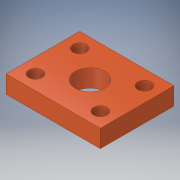
# Autodesk Inventor part: Hopper Nut Trap Holder
Saved by Autodesk Inventor 2018 (Build 220112000, 112)
## iProperties
Created: 2013-10-19
Part Number: Hopper Nut Trap Holder
Material: ABS Plastic
Document SubType Name: Modeling
Designer: Gabriel Smolnycki
Mass: 4.18388 g
Surface Area: 25.2747 cm^2
Volume: 3.94706 cm^3
Density: 1.06 g/cm^3
Appearance: Smooth - Light Orange
Sending System: SolidWorks 2017
Last Author: Gabriel Smolnycki
Last Saved: 2017-09-14
Author: Gabriel Smolnycki
Autodesk Inventor part; units mm, degrees
ref_plane "YZ Plane" through (0, 0, 0) normal (1, 0, 0) x (0, 1, 0)
ref_plane "XZ Plane" through (0, 0, 0) normal (0, 1, 0) x (-1, 0, 0)
ref_plane "XY Plane" through (0, 0, 0) normal (0, 0, 1) x (1, 0, 0)
sketch "Sketch1" plane through (0, 0, 0) normal (0, 1, 0) x (-1, 0, 0)
  line L0 (-16, 12.5) -> (-16, -12.5)
  line L1 (16, 12.5) -> (-16, 12.5)
  line L2 (16, -12.5) -> (16, 12.5)
  line L3 (-16, -12.5) -> (16, -12.5)
  constraints: 8 end point, 2 horizontal, 2 vertical
extrude "Extrusion1" add sketch "Sketch1" along normal blind 6
hole "Hole5" at (0, 6, 0) direction (0, -1, 0) diameter 10 depth 6 tip angle 118
hole "Hole4" at (-11, 6, -7.5) direction (0, -1, 0) diameter 4.5 depth 6 tip angle 118
sketch "Sketch4" plane through (0, 6, 0) normal (0, 1, 0) x (1, 0, 0)
  point P0 (11, -7.5)
hole "Hole3" at (11, 6, 7.5) direction (0, -1, 0) diameter 4.5 depth 6 tip angle 118
sketch "Sketch3" plane through (0, 6, 0) normal (0, 1, 0) x (1, 0, 0)
  point P0 (-11, 7.5)
hole "Hole2" at (11, 6, -7.5) direction (0, -1, 0) diameter 4.5 depth 6 tip angle 118
sketch "Sketch2" plane through (0, 6, 0) normal (0, 1, 0) x (1, 0, 0)
  point P0 (0, 0)
hole "Hole1" at (-11, 6, 7.5) direction (0, -1, 0) diameter 4.5 depth 6 tip angle 118
sketch "Sketch5" plane through (0, 6, 0) normal (0, 1, 0) x (1, 0, 0)
  point P0 (11, 7.5)
sketch "Sketch6" plane through (0, 6, 0) normal (0, 1, 0) x (1, 0, 0)
  point P0 (-11, -7.5)
body "Solid3"
